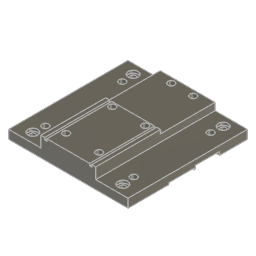
y_stage (Autodesk Fusion 360 design; units mm, degrees)
part number: 2026-04-23-15-36-49-562
Autodesk Fusion 360 part; units mm, degrees
note: some values were not read from the file. Chosen so that the rebuilt part matches the saved one: which face or edge a step refers to. Set by a fixed rule: which sketch regions a step uses.
sketch "Sketch1" plane through (0, 0, 0) normal (0, 0, 1) x (1, 0, 0)
  line L0 (-27.2, 27.2) -> (27.2, 27.2)
  line L1 (27.2, 27.2) -> (27.2, -27.2)
  line L2 (27.2, -27.2) -> (-27.2, -27.2)
  line L3 (-27.2, -27.2) -> (-27.2, 27.2)
  line L4 (-27.2, 27.2) -> (27.2, -27.2) construction
  line L5 (27.2, 27.2) -> (-27.2, -27.2) construction
  circle A0 centre (-20.1, 17.5) radius 1.5
  circle A1 centre (-20.1, -17.5) radius 1.5
  circle A2 centre (20.1, 17.5) radius 1.5
  circle A3 centre (20.1, -17.5) radius 1.5
  circle A4 centre (-4, 24.95) radius 1.5
  circle A5 centre (4, 24.95) radius 1.5
  circle A6 centre (-4, 7.95) radius 1.5
  circle A7 centre (4, 7.95) radius 1.5
  circle A8 centre (0, 10.7) radius 1.5
  dimension "d1" = 54.4
  dimension "d2" = 3
  dimension "d3" = 35
  dimension "d4" = 9.7
  dimension "d9" = 3
  dimension "d10" = 24.95
  dimension "d11" = 4
  dimension "d12" = 4
  dimension "d19" = 7.1
  dimension "d20" = 7.1
  dimension "d21" = 17
  dimension "d22" = 16.5
  dimension "d23" = 3
  constraint horizontal L0
  constraint perpendicular L0 L1
  constraint parallel L0 L2
  constraint parallel L1 L3
  constraint coincident L4 origin
  constraint coincident L5 origin
  constraint equal L0 L3
  constraint vertical A0.centre A1.centre
  constraint horizontal A1.centre A3.centre
  constraint vertical A2.centre A3.centre
  constraint horizontal A0.centre A2.centre
  constraint equal A0 A1
  constraint equal A1 A3
  constraint equal A2 A3
  constraint equal A4 A5
  constraint horizontal A4.centre A5.centre
  constraint vertical A5.centre A7.centre
  constraint vertical A4.centre A6.centre
  constraint equal A4 A6
  constraint equal A6 A7
  constraint horizontal A6.centre A7.centre
  constraint vertical origin A8.centre
  measures "d1" distance of L0.start L0.end
  measures "d2" diameter of A0
  measures "d3" distance of A0.centre A1.centre
  measures "d4" distance of L0 A0.centre
  measures "d9" diameter of A4
  measures "d10" vertical distance of origin A4.centre
  measures "d11" horizontal distance of origin A4.centre
  measures "d12" horizontal distance of origin A5.centre
  measures "d19" distance of L3 A0.centre
  measures "d20" distance of L1 A2.centre
  measures "d21" distance of A4.centre A6.centre
  measures "d22" distance of L0 A8.centre
  measures "d23" diameter of A8
extrude "Extrude1" add sketch "Sketch1" along normal blind 4 contours L0 L1 L2 L3 | A4 | A5 | A6 | A7 | A8
sketch "Sketch2" plane through (0, 0, 4) normal (0, 0, 1) x (-1, 0, 0)
  circle A0 centre (-20.1, 17.5) radius 1.5
  circle A1 centre (20.1, -17.5) radius 1.5
  circle A2 centre (20.1, 17.5) radius 1.5
  circle A3 centre (-20.1, -17.5) radius 1.5
  line L0 (27.2, 27.2) -> (-27.2, 27.2)
  line L1 (-27.2, 27.2) -> (-27.2, -27.2)
  line L2 (-27.2, -27.2) -> (27.2, -27.2)
  line L3 (27.2, -27.2) -> (27.2, 27.2)
  line L4 (12.5, -27.2) -> (-12.5, -27.2)
  line L5 (-12.5, -27.2) -> (-12.5, 27.2)
  line L6 (-12.5, 27.2) -> (12.5, 27.2)
  line L7 (12.5, 27.2) -> (12.5, -27.2)
  line L8 (12.5, -27.2) -> (-12.5, 27.2) construction
  line L9 (-12.5, -27.2) -> (12.5, 27.2) construction
  dimension "d13" = 25
  constraint horizontal L4
  constraint perpendicular L4 L5
  constraint parallel L4 L6
  constraint parallel L5 L7
  constraint coincident L8 origin
  constraint coincident L9 origin
  constraint coincident L2 L4.start
  measures "d13" distance of L4.start L4.end
extrude "Extrude2" add sketch "Sketch2" along normal blind 3 contours L0 L2 L4 L5 L6 L7
sketch "Sketch5" plane through (0, 0, 7) normal (0, 0, 1) x (-1, 0, 0)
  line L0 (12.5, 27.2) -> (-12.5, 27.2)
  line L1 (-12.5, 27.2) -> (-12.5, -27.2)
  line L2 (-12.5, -27.2) -> (12.5, -27.2)
  line L3 (12.5, -27.2) -> (12.5, 27.2)
  circle A0 centre (7.5, -0.3) radius 1.5
  circle A1 centre (-7.5, -0.3) radius 1.5
  circle A2 centre (7.5, 20.7) radius 1.5
  circle A3 centre (-7.5, 20.7) radius 1.5
  circle A4 centre (5, -24.7) radius 1.5
  circle A5 centre (-5, -24.7) radius 1.5
  circle A6 centre (5, -10.7) radius 1.5
  circle A7 centre (-5, -10.7) radius 1.5
  dimension "d27" = 15
  dimension "d28" = 21
  dimension "d29" = 3
  dimension "d31" = 7.5
  dimension "d34" = 10
  dimension "d35" = 14
  dimension "d36" = 3
  dimension "d37" = 5
  dimension "d38" = 2.5
  dimension "d49" = 26.9
  constraint vertical A0.centre A2.centre
  constraint horizontal A0.centre A1.centre
  constraint horizontal A2.centre A3.centre
  constraint vertical A1.centre A3.centre
  constraint equal A2 A3
  constraint equal A0 A2
  constraint equal A0 A1
  constraint vertical A4.centre A6.centre
  constraint horizontal A6.centre A7.centre
  constraint vertical A5.centre A7.centre
  constraint horizontal A4.centre A5.centre
  constraint equal A4 A5
  constraint equal A5 A7
  constraint equal A6 A7
  measures "d27" distance of A0.centre A1.centre
  measures "d28" distance of A0.centre A2.centre
  measures "d29" diameter of A0
  measures "d31" horizontal distance of origin A2.centre
  measures "d34" distance of A4.centre A5.centre
  measures "d35" vertical distance of A4.centre A6.centre
  measures "d36" diameter of A4
  measures "d37" horizontal distance of origin A4.centre
  measures "d38" distance of L2 A4.centre
  measures "d49" distance of L2 A0.centre
extrude "Extrude5" cut sketch "Sketch5" against normal blind 3 contours A0 | A1 | A2 | A3 | A4 | A5
sketch "Sketch6" plane through (0, 0, 7) normal (0, 0, 1) x (-1, 0, 0)
  line L0 (12.5, 27.2) -> (-12.5, 27.2)
  line L1 (-12.5, 27.2) -> (-12.5, -27.2)
  line L2 (-12.5, -27.2) -> (12.5, -27.2)
  line L3 (12.5, -27.2) -> (12.5, 27.2)
  circle A0 centre (5, -24.7) radius 1.5
  circle A1 centre (7.5, 20.7) radius 1.5
  circle A2 centre (7.5, -0.3) radius 1.5
  circle A3 centre (-5, -24.7) radius 1.5
  circle A4 centre (-7.5, 20.7) radius 1.5
  circle A5 centre (-7.5, -0.3) radius 1.5
  line L4 (12.5, 27.2) -> (-12.5, 27.2)
  line L5 (-12.5, 27.2) -> (-12.5, -2.3)
  line L6 (-12.5, -2.3) -> (12.5, -2.3)
  line L7 (12.5, -2.3) -> (12.5, 27.2)
  dimension "d39" = 29.5
  constraint horizontal L4
  constraint vertical L5
  constraint horizontal L6
  constraint vertical L7
  constraint coincident L1 L5.end
  constraint coincident L0.start L3.end
  measures "d39" distance of L0.start L6.end
extrude "Extrude6" add sketch "Sketch6" along normal blind 2 contours L0 L1 L3 L4 L5 L6 L7
extrude "Extrude8" add 1 faces at (1.484, 9.3012, 7) along direction (0, 0, 1) blind 0.3
sketch "Sketch8" plane through (0, 0, 9) normal (0, 0, 1) x (-1, 0, 0)
  circle A0 centre (7.5, -0.3) radius 1.5
  circle A1 centre (7.5, 20.7) radius 1.5
  circle A2 centre (-7.5, 20.7) radius 1.5
  circle A3 centre (-7.5, -0.3) radius 1.5
  line L0 (12.5, -2.3) -> (12.5, 27.2)
  line L1 (12.5, 27.2) -> (-12.5, 27.2)
  line L2 (-12.5, 27.2) -> (-12.5, -2.3)
  line L3 (-12.5, -2.3) -> (12.5, -2.3)
  line L4 (10.73, -2.3) -> (9.73, -2.3)
  line L5 (9.73, -2.3) -> (9.73, 27.2)
  line L6 (9.73, 27.2) -> (10.73, 27.2)
  line L7 (10.73, 27.2) -> (10.73, -2.3)
  line L8 (-9.73, -2.3) -> (-10.73, -2.3)
  line L9 (-10.73, -2.3) -> (-10.73, 27.2)
  line L10 (-10.73, 27.2) -> (-9.73, 27.2)
  line L11 (-9.73, 27.2) -> (-9.73, -2.3)
  dimension "d52" = 1
  dimension "d53" = 1.77
  dimension "d54" = 1.77
  constraint horizontal L4
  constraint vertical L5
  constraint horizontal L6
  constraint vertical L7
  constraint coincident L1 L5.end
  constraint coincident L3 L4.start
  constraint horizontal L8
  constraint vertical L9
  constraint horizontal L10
  constraint vertical L11
  constraint coincident L1 L9.end
  constraint coincident L3 L8.start
  constraint equal L4 L8
  measures "d52" distance of L4.start L4.end
  measures "d53" distance of L0 L7
  measures "d54" distance of L2 L9
extrude "Extrude9" cut sketch "Sketch8" against normal blind 1 contours L1 L3 L4 L5 L6 L7 | L1 L3 L8 L9 L10 L11
sketch "Sketch9" plane through (0, 0, 0) normal (0, 0, -1) x (1, 0, 0)
  circle A0 centre (20.1, 17.5) radius 1.5
  circle A1 centre (-20.1, 17.5) radius 1.5
  circle A2 centre (20.1, -17.5) radius 1.5
  circle A3 centre (-20.1, -17.5) radius 1.5
  line L0 (27.2, 27.2) -> (-27.2, 27.2)
  line L1 (-27.2, 27.2) -> (-27.2, -27.2)
  line L2 (-27.2, -27.2) -> (27.2, -27.2)
  line L3 (27.2, -27.2) -> (27.2, 27.2)
  circle A4 centre (-20.5, 22.85) radius 1.25
  circle A5 centre (20.5, 22.85) radius 1.25
  circle A6 centre (-20.5, -22.85) radius 1.25
  circle A7 centre (20.5, -22.85) radius 1.25
  dimension "d57" = 41
  dimension "d58" = 45.7
  dimension "d59" = 2.5
  dimension "d60" = 20.5
  dimension "d61" = 22.85
  constraint equal A6 A7
  constraint equal A4 A6
  constraint equal A4 A5
  constraint horizontal A4.centre A5.centre
  constraint vertical A5.centre A7.centre
  constraint horizontal A6.centre A7.centre
  constraint vertical A4.centre A6.centre
  measures "d57" distance of A4.centre A5.centre
  measures "d58" distance of A4.centre A6.centre
  measures "d59" diameter of A6
  measures "d60" horizontal distance of origin A6.centre
  measures "d61" vertical distance of origin A4.centre
extrude "Extrude10" cut sketch "Sketch9" against normal blind 5 contours A4 | A5 | A6 | A7
sketch "Sketch10" plane through (0, 0, 4) normal (0, 0, 1) x (-1, 0, 0)
  circle A0 centre (20.5, 22.85) radius 1.25
  circle A1 centre (20.5, -22.85) radius 1.25
  line L0 (12.5, 27.2) -> (12.5, -27.2)
  line L1 (12.5, -27.2) -> (27.2, -27.2)
  line L2 (27.2, -27.2) -> (27.2, 27.2)
  line L3 (27.2, 27.2) -> (12.5, 27.2)
  circle A2 centre (20.1, 17.5) radius 1.5
  circle A3 centre (20.1, -17.5) radius 1.5
  circle A4 centre (20.5, -22.85) radius 2.25
  circle A5 centre (20.5, 22.85) radius 2.25
  circle A6 centre (-20.5, 22.85) radius 2.25
  circle A7 centre (-20.5, 22.85) radius 1.25
  circle A8 centre (-20.5, -22.85) radius 2.25
  circle A9 centre (-20.5, -22.85) radius 1.25
  dimension "d64" = 4.5
  constraint concentric A1 A4
  constraint concentric A0 A5
  constraint concentric A6 A7
  constraint concentric A8 A9
  constraint equal A5 A6
  constraint equal A4 A6
  constraint equal A4 A8
  measures "d64" diameter of A8
extrude "Extrude11" cut sketch "Sketch10" against normal blind 1.15 contours A4 | A5 | A6 | A8
sketch "Sketch11" plane through (0, 0, 0) normal (0, 0, -1) x (1, 0, 0)
  line L0 (27.2, 27.2) -> (-27.2, 27.2)
  line L1 (-27.2, 27.2) -> (-27.2, -27.2)
  line L2 (-27.2, -27.2) -> (27.2, -27.2)
  line L3 (27.2, -27.2) -> (27.2, 27.2)
  circle A0 centre (-20.1, -17.5) radius 1.5
  circle A1 centre (20.1, -17.5) radius 1.5
  circle A2 centre (-20.1, 17.5) radius 1.5
  circle A3 centre (20.1, 17.5) radius 1.5
  circle A4 centre (20.5, -22.85) radius 1.25
  circle A5 centre (-20.5, -22.85) radius 1.25
  circle A6 centre (20.5, 22.85) radius 1.25
  circle A7 centre (-20.5, 22.85) radius 1.25
  line L4 (-27.2, -14.5) -> (27.2, -14.5)
  line L5 (27.2, -14.5) -> (27.2, -3.5)
  line L6 (27.2, -3.5) -> (-27.2, -3.5)
  line L7 (-27.2, -3.5) -> (-27.2, -14.5)
  dimension "d67" = 11
  dimension "d68" = 12.7
  constraint horizontal L4
  constraint vertical L5
  constraint horizontal L6
  constraint vertical L7
  constraint coincident L3 L5.end
  constraint coincident L1 L4.start
  measures "d67" distance of L4.start L6.end
  measures "d68" distance of L2 L4
extrude "Extrude12" cut sketch "Sketch11" against normal blind 1.6 contours L1 L3 L4 L5 L6 L7
sketch "Sketch12" plane through (0, 0, 0) normal (0, 0, -1) x (1, 0, 0)
  line L0 (-27.2, -3.5) -> (27.2, -3.5)
  line L1 (27.2, -3.5) -> (27.2, 27.2)
  line L2 (27.2, 27.2) -> (-27.2, 27.2)
  line L3 (-27.2, 27.2) -> (-27.2, -3.5)
  circle A0 centre (-20.5, 22.85) radius 1.25
  circle A1 centre (20.5, 22.85) radius 1.25
  circle A2 centre (20.1, 17.5) radius 1.5
  circle A3 centre (-20.1, 17.5) radius 1.5
  line L4 (27.2, -3) -> (-27.2, -3)
  line L5 (-27.2, -3) -> (-27.2, 8.5)
  line L6 (-27.2, 8.5) -> (27.2, 8.5)
  line L7 (27.2, 8.5) -> (27.2, -3)
  line L8 (-27.2, -27.2) -> (27.2, -27.2)
  dimension "d71" = 11.5
  dimension "d72" = 24.2
  constraint horizontal L4
  constraint vertical L5
  constraint horizontal L6
  constraint vertical L7
  constraint coincident L3 L5.end
  constraint coincident L1 L4.start
  measures "d71" distance of L4.start L6.end
  measures "d72" distance of L4 L8
extrude "Extrude13" cut sketch "Sketch12" against normal blind 0.8 contours L1 L3 L4 L5 L6 L7
ref_plane "WorkPlane1" through (0, 0, 1.5) normal (-1, 0, 0) x (0, -1, 0)
sketch "Sketch7" plane through (0, 0, 0) normal (-1, 0, 0) x (0, -1, 0)
  line L0 (27.2, 0) -> (27.2, 8.1)
  line L1 (27.2, 8.1) -> (17.2, 8.1)
  line L2 (17.2, 8.1) -> (9.1, 0)
  line L3 (9.1, 0) -> (27.2, 0)
  line L4 (-2.3, 8.1) -> (27.2, 8.1)
  line L5 (27.2, 3) -> (12.1, 3)
  line L6 (12.1, 3) -> (12.1, 0)
  point P0 (27.2, 8.1)
  point P1 (27.2, 0)
  dimension "d42" = 10
  dimension "d43" = 45
  dimension "d46" = 3
  constraint vertical L0
  constraint perpendicular L0 L1
  constraint horizontal L3
  constraint coincident P0 L0.end
  constraint coincident L0.start L3.end
  constraint coincident L0 L5.start
  constraint coincident L2 L5.end
  constraint perpendicular L0 L5
  constraint coincident L3 L6.end
  constraint perpendicular L3 L6
  measures "d42" distance of P0 L1.end
  measures "d43" angle of L2 L4
  measures "d46" distance of L3 L5
extrude "Extrude7" [suppressed]
sketch "Sketch4" plane through (0, 0, 0) normal (0, 0, -1) x (1, 0, 0)
  circle A0 centre (20.4, 17.5) radius 1.5
  circle A1 centre (0, -11) radius 1.5
  circle A2 centre (-5, -9.3) radius 1.5
  circle A3 centre (5, -9.3) radius 1.5
  circle A4 centre (-20.4, -17.5) radius 1.5
  circle A5 centre (20.4, -17.5) radius 1.5
  circle A6 centre (-5, -25) radius 1.5
  circle A7 centre (5, -25) radius 1.5
  line L0 (27.5, 27.5) -> (-27.5, 27.5)
  line L1 (-27.5, 27.5) -> (-27.5, -27.5)
  line L2 (-27.5, -27.5) -> (27.5, -27.5)
  line L3 (27.5, -27.5) -> (27.5, 27.5)
  circle A8 centre (-20.4, 17.5) radius 1.5
  circle A9 centre (0, -11) radius 2.5
  dimension "d24" = 5
  constraint concentric A1 A9
  measures "d24" diameter of A9
extrude "Extrude4" [suppressed]
sketch "Sketch3" plane through (0, 0, 6) normal (0, 0, 1) x (-1, 0, 0)
  circle A0 centre (-5, -20) radius 1.5
  circle A1 centre (5, -20) radius 1.5
  line L0 (10.3, 25) -> (-10.3, 25)
  line L1 (-10.3, 25) -> (-10.3, -25)
  line L2 (-10.3, -25) -> (10.3, -25)
  line L3 (10.3, -25) -> (10.3, 25)
  line L4 (10.3, 25) -> (-10.3, 25)
  line L5 (-10.3, 25) -> (-10.3, 20)
  line L6 (-10.3, 20) -> (10.3, 20)
  line L7 (10.3, 20) -> (10.3, 25)
  dimension "d16" = 5
  constraint horizontal L4
  constraint vertical L5
  constraint horizontal L6
  constraint vertical L7
  constraint coincident L1 L5.end
  constraint coincident L0.start L3.end
  measures "d16" distance of L0.end L5.end
extrude "Extrude3" [suppressed]
equation "d4 = ( d1 - d3 ) / 2"
equation "d5 = 26 mm + 1.9 mm - 2.5 mm"
equation "d10 = 25 mm - 0.95 mm + 1.2 mm - 0.3 mm"
equation "d12 = d11"
equation "d19 = d20"
equation "d22 = 14 mm + 2.5 mm"
equation "d23 = d9"
equation "d31 = d27 / 2"
equation "d37 = d34 / 2"
equation "d60 = d57 / 2"
equation "d61 = d58 / 2"
